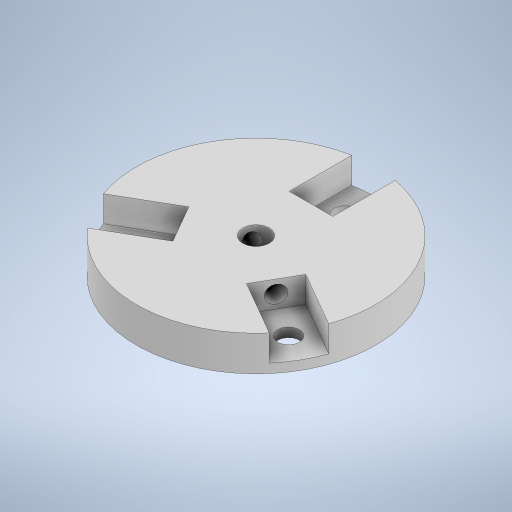
# Autodesk Inventor part: 1. housing hub
Saved by Autodesk Inventor 2024 (Build 280153000, 153)
## iProperties
Created: 2024-06-08
Part Number: 1. housing hub
Material: Generic
Document SubType Name: Sheet Metal
Designer: albah
Density: 1 g/cm^3
Sheet Metal Rule: Default_mm
Appearance: Default
Author: albah
Autodesk Inventor part; units mm, degrees
ref_plane "YZ Plane" through (0, 0, 0) normal (1, 0, 0) x (0, 1, 0)
ref_plane "XZ Plane" through (0, 0, 0) normal (0, 1, 0) x (-1, 0, 0)
ref_plane "XY Plane" through (0, 0, 0) normal (0, 0, 1) x (1, 0, 0)
sketch "Sketch1" plane through (0, 0, 0) normal (0, 1, 0) x (-1, 0, 0)
  circle A0 centre (0, 0) radius 27.5
  circle A1 centre (0, 0) radius 3.05
  dimension "d0" = 55
  dimension "d1" = 6.1
  constraints: 2 centre point, 2 coincident
  measures "d0" diameter of A0
  measures "d1" diameter of A1
extrude "Extrusion1" add sketch "Sketch1" along normal blind 8.1
sketch "Sketch2" plane through (0, 8.1, 0) normal (0, 1, 0) x (1, 0, 0)
  circle A0 centre (0, 0) radius 27.5 projected
  circle A1 centre (0, 0) radius 3.05 projected
  line L0 (0, 0) -> (0, 27.5)
  line L1 (-5, 42.3445) -> (5, 42.3445)
  line L2 (5, 42.3445) -> (5, 12.6555)
  line L3 (5, 12.6555) -> (-5, 12.6555)
  line L4 (-5, 12.6555) -> (-5, 42.3445)
  line L5 (-5, 42.3445) -> (5, 12.6555) construction
  line L6 (5, 42.3445) -> (-5, 12.6555) construction
  line L7 (-39.1714, -16.8421) -> (-13.46, -1.9976)
  line L8 (-13.46, -1.9976) -> (-8.46, -10.6579)
  line L9 (-8.46, -10.6579) -> (-34.1714, -25.5024)
  line L10 (34.1714, -25.5024) -> (8.46, -10.6579)
  line L11 (8.46, -10.6579) -> (13.46, -1.9976)
  line L12 (13.46, -1.9976) -> (39.1714, -16.8421)
  point P0 (-25.9187, -9.1907)
  point P1 (-20.9187, -17.8509)
  point P2 (20.9187, -17.8509)
  point P3 (25.9187, -9.1907)
  dimension "d7" = 360
  constraints: 26 end point, 2 midpoint, 2 parallel, 1 horizontal, 1 perpendicular, 1 vertical, 24 other
extrude "Extrusion2" cut sketch "Sketch2" against normal blind 6 contours L2 L3 L0 A0 | A0 L4 L1 L2 | A0 L10 L11 L12 | L0 L3 L4 A0 | A0 L7 L8 L9
sketch "Sketch3" plane through (8.46, 2.1, 10.6579) normal (0.8660254, 0, 0.5) x (0.5, 0, -0.8660254)
  circle A0 centre (5, 3) radius 1.75
  point P0 (5, -2.1)
  dimension "d11" = 3.5
  constraints: 1 centre point
  measures "d11" diameter of A0
extrude "Extrusion3" cut sketch "Sketch3" against normal through all
sketch "Sketch4" plane through (8.46, 2.1, 10.6579) normal (0.8660254, 0, 0.5) x (0.5, 0, -0.8660254)
  circle A0 centre (5, 3) radius 1.75 projected
  circle A1 centre (5, 3) radius 2
  point P0 (5, -2.1)
  dimension "d14" = 4
  constraints: 1 centre point, 1 coincident
  measures "d14" diameter of A1
extrude "Extrusion4" cut sketch "Sketch4" against normal blind 5 contours A0 | A1
sketch "Sketch5" plane through (0, 8.1, 0) normal (0, 1, 0) x (1, 0, 0)
  circle A0 centre (0, 0) radius 20.4686
  circle A1 centre (0, 20.4686) radius 2.5
  circle A2 centre (-17.7264, -10.2343) radius 2.5
  circle A3 centre (0, 0) radius 20.4686
  circle A4 centre (17.7264, -10.2343) radius 2.5
  circle A5 centre (0, 0) radius 20.4686
  dimension "d17" = 5
  dimension "d20" = 360
  constraints: 3 centre point, 1 coincident, 1 vertical alignment, 21 other
  measures "d17" diameter of A1
extrude "Extrusion5" cut sketch "Sketch5" against normal through all contours A1 A0 | A0 A1 | A4 A0 | A0 A4 | A2 A0 | A0 A2
equation "\"BendRadius\" = Thickness"
equation "\"BendReliefWidth\" = Thickness"
equation "\"BendReliefDepth\" = 0.5 * Thickness"
equation "\"CornerReliefSize\" = 4 * Thickness"
equation "\"MinimumRemnant\" = 2 * Thickness"
equation "\"TransitionRadius\" = BendRadius"
equation "\"JacobiRadiusSize\" = BendRadius"
equation "\"GapSize\" = Thickness"
equation "\"Thickness\" = 0.5"
body "Solid1"
